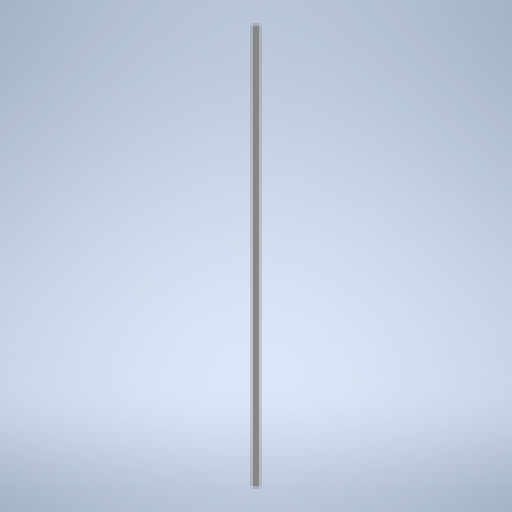
# Autodesk Inventor part: Stangeschaufelrad
Saved by Autodesk Inventor 2024.4 (Build 284460000, 460)
## iProperties
Created: 2026-01-14
Part Number: Stangeschaufelrad
Material: Edelstahl
Description: Stangeschaufelrad
Document SubType Name: Modeling
Designer: Philf
Mass: 3342.65 g
Surface Area: 841.947 cm^2
Volume: 417.832 cm^3
Density: 8 g/cm^3
Appearance: Halbpoliert
Masse[kg]: 0,754 kg
Autodesk Inventor part; units mm, degrees
ref_plane "YZ Plane" through (0, 0, 0) normal (1, 0, 0) x (0, 1, 0)
ref_plane "XZ Plane" through (0, 0, 0) normal (0, 1, 0) x (-1, 0, 0)
ref_plane "XY Plane" through (0, 0, 0) normal (0, 0, 1) x (1, 0, 0)
sketch "Skizze1" plane through (0, 0, 0) normal (0, 0, 1) x (1, 0, 0)
  circle A0 centre (0, 0) radius 10
  dimension "d0" = 20
  constraints: 1 centre point, 1 coincident
  measures "d0" diameter of A0
extrude "Extrusion1" add sketch "Skizze1" along normal blind 1330
